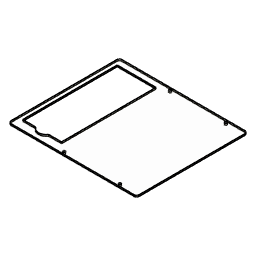
silvia_tray (Autodesk Fusion 360 design; units mm, degrees)
Autodesk Fusion 360 part; units mm, degrees
sketch "Top Panel" plane through (0, 0, 0) normal (0, 0, 1) x (1, 0, 0)
  line L0 (5.15, 228.5) -> (259.15, 228.5)
  line L1 (264.15, 223.5) -> (264.15, 5)
  line L2 (259.15, 0) -> (5.15, 0)
  line L3 (0.15, 5) -> (0.15, 223.5)
  line L4 (10.15, 214) -> (90, 214)
  line L5 (90, 214) -> (90, 19.5)
  line L6 (10.15, 19.5) -> (10.15, 214)
  line L7 (50.075, 27.7654) -> (10.15, 27.7654) construction
  line L8 (50.075, 27.7654) -> (90, 27.7654) construction
  line L9 (50.075, 27.7654) -> (50.075, 12) construction
  arc A0 (36.65, 19.5) -> (63.323, 19.5) centre (49.9865, 27.7752) ccw
  arc A1 (264.15, 223.5) -> (259.15, 228.5) centre (259.15, 223.5) ccw
  arc A2 (259.15, 0) -> (264.15, 5) centre (259.15, 5) ccw
  arc A3 (0.15, 5) -> (5.15, 0) centre (5.15, 5) ccw
  arc A4 (5.15, 228.5) -> (0.15, 223.5) centre (5.15, 223.5) ccw
  circle A5 centre (109.65, 5.1) radius 2.5
  line L10 (109.65, 5.1) -> (107.15, 5.1) construction
  line L11 (109.65, 5.1) -> (109.65, 2.6) construction
  line L12 (109.65, 2.6) -> (109.65, 0) construction
  line L13 (107.15, 5.1) -> (0.15, 5.1) construction
  circle A6 centre (224.65, 5.1) radius 2.5
  line L14 (224.65, 5.1) -> (227.15, 5.1) construction
  line L15 (224.65, 2.6) -> (224.65, 5.1) construction
  line L16 (224.65, 2.6) -> (224.65, 0) construction
  line L17 (227.15, 5.1) -> (264.15, 5.1) construction
  circle A7 centre (109.65, 223.4) radius 2.5
  circle A8 centre (224.65, 223.4) radius 2.5
  line L18 (109.65, 223.4) -> (107.15, 223.4) construction
  line L19 (109.65, 223.4) -> (109.65, 225.9) construction
  line L20 (107.15, 223.4) -> (0.15, 223.4) construction
  line L21 (224.65, 223.4) -> (224.65, 225.9) construction
  line L22 (224.65, 223.4) -> (227.15, 223.4) construction
  line L23 (224.65, 225.9) -> (224.65, 228.5) construction
  line L24 (227.15, 223.4) -> (264.15, 223.4) construction
  line L25 (109.65, 225.9) -> (109.65, 228.5) construction
  line L26 (90, 19.5) -> (63.323, 19.5)
  line L27 (36.65, 19.5) -> (10.15, 19.5)
  point P0 (36.65, 19.5)
  dimension "d1" = 264
  dimension "d2" = 228.5
  dimension "d3" = 79.85
  dimension "d4" = 10
  dimension "d6" = 14.5
  dimension "d8" = 12
  dimension "d9" = 26.5
  dimension "d10" = 5
  dimension "d17" = 2.6
  dimension "d18" = 107
  dimension "d19" = 2.5
  dimension "d20" = 37
  constraint horizontal L0
  constraint vertical L1
  constraint horizontal L2
  constraint vertical L3
  constraint horizontal L4
  constraint vertical L5
  constraint vertical L6
  constraint coincident L6 L7.end
  constraint perpendicular L6 L7
  constraint coincident L5 L8.end
  constraint perpendicular L5 L8
  constraint equal L7 L8
  constraint perpendicular L8 L9
  constraint coincident P0 A0.start
  constraint tangent L0 A1
  constraint tangent L1 A1
  constraint tangent L1 A2
  constraint tangent L2 A2
  constraint equal A1 A2
  constraint tangent L2 A3
  constraint tangent L3 A3
  constraint equal A2 A3
  constraint tangent L0 A4
  constraint tangent L3 A4
  constraint equal A1 A4
  constraint coincident A5.centre L10.start
  constraint coincident A5 L10.end
  constraint perpendicular L5 L10
  constraint coincident A5 L11.end
  constraint perpendicular L10 L11
  constraint coincident L2 L12.end
  constraint perpendicular L2 L12
  constraint coincident L3 L13.end
  constraint horizontal L13
  constraint coincident A6.centre L14.start
  constraint coincident A6 L14.end
  constraint horizontal L14
  constraint coincident A6 L15.start
  constraint perpendicular L14 L15
  constraint coincident L2 L16.end
  constraint perpendicular L2 L16
  constraint coincident L1 L17.end
  constraint perpendicular L1 L17
  constraint equal L10 L14
  constraint equal L12 L16
  constraint coincident A7.centre L18.start
  constraint coincident A7 L18.end
  constraint perpendicular L1 L18
  constraint coincident A7 L19.end
  constraint perpendicular L18 L19
  constraint coincident L3 L20.end
  constraint perpendicular L3 L20
  constraint coincident A8.centre L21.start
  constraint coincident A8 L21.end
  constraint perpendicular L20 L21
  constraint coincident A8 L22.end
  constraint perpendicular L21 L22
  constraint coincident L0 L23.end
  constraint perpendicular L0 L23
  constraint coincident L1 L24.end
  constraint perpendicular L1 L24
  constraint equal L17 L24
  constraint equal L10 L18
  constraint coincident L0 L25.end
  constraint perpendicular L0 L25
  constraint equal L12 L25
  constraint equal L10 L22
  constraint equal L12 L23
  constraint equal L13 L20
  constraint perpendicular L5 L26
  constraint perpendicular L6 L27
  measures "d1" distance of L1 L3
  measures "d2" distance of L0 L2
  measures "d3" distance of L5 L6
  measures "d4" distance of L3 L6
  measures "d6" distance of L0 L4
  measures "d8" distance of L2 L9.end
  measures "d9" distance of L6 P0
  measures "d10" radius of A1
  measures "d17" distance of L11.end L12.end
  measures "d18" distance of L10.end L13.end
  measures "d19" distance of A5.centre L10.end
  measures "d20" distance of L14.end L17.end
extrude "Extrude1" add sketch "Top Panel" along normal blind 3
named bodies: "Top Panel"
